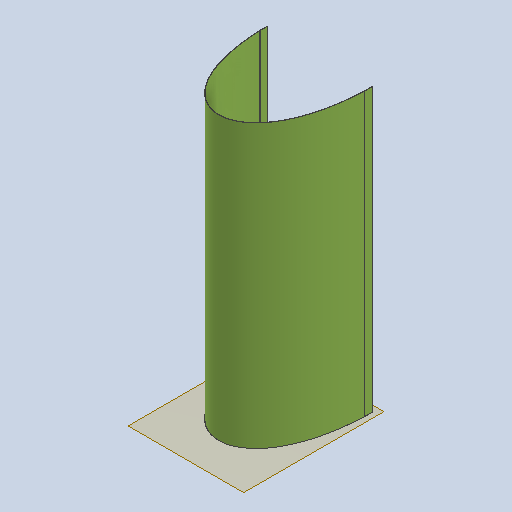
# Autodesk Inventor part: canvas-cover-deployed
Saved by Autodesk Inventor 2023 (Build 270158030, 158C)
## iProperties
Created: 2024-09-25
Part Number: canvas-cover-deployed
Material: Generic
Document SubType Name: Modeling
Designer: Imogen Heard
Density: 1 g/cm^3
Appearance: Default
Author: Imogen Heard
Autodesk Inventor part; units mm, degrees
ref_plane "YZ Plane" through (0, 0, 0) normal (1, 0, 0) x (0, 1, 0)
ref_plane "XZ Plane" through (0, 0, 0) normal (0, 1, 0) x (-1, 0, 0)
ref_plane "XY Plane" through (0, 0, 0) normal (0, 0, 1) x (1, 0, 0)
ref_plane "Work Plane1" through (76.6258, 25, 425) normal (-0.0000002, 1, 0) x (1, 0.0000002, 0)
sketch "Sketch1" plane through (76.6258, 25, 425) normal (-0.0000002, 1, 0) x (1, 0.0000002, 0)
  spline S0 degree 4 poles (-350, 375) (-320, -275) (0, -425) (320, -275) (350, 375) knots 1 1 1 1 1 2 2 2 2 2 projected
  line L0 (350, 375) -> (347.9979, 375)
  line L1 (347.9979, 375) -> (347.9979, 425)
  line L2 (347.9979, 425) -> (350, 425)
  line L3 (350, 425) -> (350, 375)
  line L4 (-347.9979, 375) -> (-350, 375)
  line L5 (-350, 375) -> (-350, 425)
  line L6 (-350, 425) -> (-347.9979, 425)
  line L7 (-347.9979, 425) -> (-347.9979, 375)
  line L8 (350, 425) -> (-350, 425) projected
  spline S1 degree 5 poles (-347.9979, 375) (-346.0284, 332.3773) (-342.7984, 289.8122) (-338.1422, 247.3651) (-326.7683, 170.9664) (-309.046, 95.8136) (-299.6921, 62.5697) (-279.8558, 3.4629) (-253.7566, -53.1178) (-240.7312, -77.6833) (-214.2698, -120.6219) (-182.0256, -159.3421) (-166.3213, -175.6301) (-134.7805, -203.1852) (-98.784, -224.4736) (-81.3473, -232.6678) (-46.0767, -244.8104) (-9.0446, -249.0034) (9.0446, -249.0034) (46.0767, -244.8104) (81.3473, -232.6678) (98.784, -224.4736) (134.7805, -203.1852) (166.3213, -175.6301) (182.0256, -159.3421) (214.2698, -120.6219) (240.7312, -77.6833) (253.7566, -53.1178) (279.8558, 3.4629) (299.6921, 62.5697) (309.046, 95.8136) (326.7683, 170.9664) (338.1422, 247.3651) (342.7984, 289.8122) (346.0284, 332.3773) (347.9979, 375) knots 0 0 0 0 0 0 0.137161 0.137161 0.137161 0.248035 0.248035 0.248035 0.337224 0.337224 0.337224 0.409677 0.409677 0.409677 0.471186 0.471186 0.471186 0.528814 0.528814 0.528814 0.590323 0.590323 0.590323 0.662776 0.662776 0.662776 0.751965 0.751965 0.751965 0.862839 0.862839 0.862839 1 1 1 1 1 1
  point P0 (-76.6258, 425)
  dimension "d0" = 2
  constraints: 16 end point, 4 parallel, 2 horizontal, 2 perpendicular, 1 horizontal alignment, 2 other
ref_plane "Work Plane2" through (-283.6242, 1904.9999, -0.2055) normal (0.0000002, -1, 0) x (1, 0.0000002, 0)
extrude "Extrusion1" add sketch "Sketch1" along normal up to surface (1880 mm away) contours L4 S1 L0 S0 | L5 L6 L7 L4 | L0 L1 L2 L3
